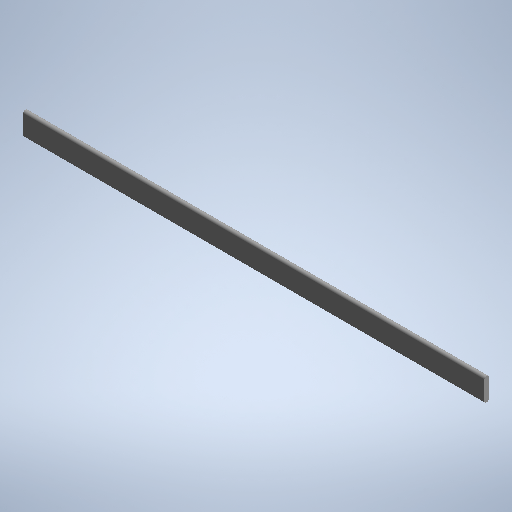
# Autodesk Inventor part: CFSTRIP-2-12-2
Saved by Autodesk Inventor 2025.4 (Build 294407000, 407)
## iProperties
Created: 2026-04-27
Part Number: CFSTRIP-2-12-2
Material: Générique
Document SubType Name: Modeling
Designer: louis
Density: 1 g/cm^3
Appearance: Par défaut
Author: louis
Autodesk Inventor part; units mm, degrees
ref_plane "YZ Plane" through (0, 0, 0) normal (1, 0, 0) x (0, 1, 0)
ref_plane "XZ Plane" through (0, 0, 0) normal (0, 1, 0) x (-1, 0, 0)
ref_plane "XY Plane" through (0, 0, 0) normal (0, 0, 1) x (1, 0, 0)
sketch "Sketch2" plane through (0, 0, 0) normal (1, 0, 0) x (0, 1, 0)
  line L0 (0, -4) -> (0, 4) construction
  line L1 (1, -4) -> (1, 4)
  line L2 (-1, 4) -> (-1, -4)
  arc A0 (-1, -4) -> (1, -4) centre (0, -4) ccw
  arc A1 (1, 4) -> (-1, 4) centre (0, 4) ccw
  point P0 (0, 0)
  point P1 (0, -5)
  point P2 (0, 5)
  dimension "d1" = 2
  dimension "d2" = 10
  constraints: 8 end point, 6 point on circle, 4 tangent, 2 centre point, 1 midpoint, 1 parallel, 1 vertical
  measures "d1" diameter of A1
  measures "d2" distance of point (0, -5) point (0, 5)
extrude "Extrusion1" add sketch "Sketch2" along normal mid plane 200
body "Solid1"
